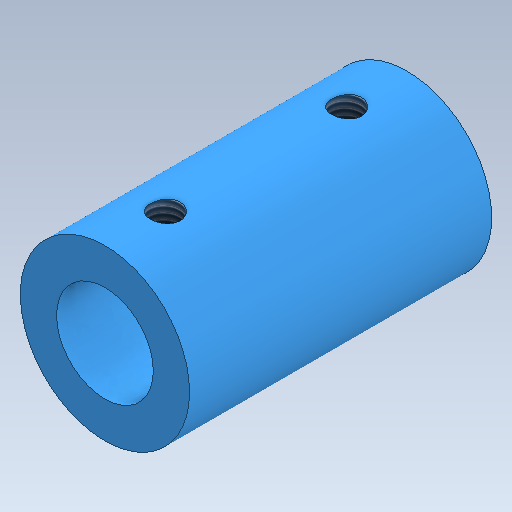
# Autodesk Inventor part: 10-03-05 Hub
Saved by Autodesk Inventor 2020 (Build 240168000, 168)
## iProperties
Created: 2019-10-05
Part Number: 10-03-05 Hub
Material: Generic
Document SubType Name: Modeling
Designer: iuliu
Density: 1 g/cm^3
Appearance: Default(1)
Author: iuliu
Subject: 005
Autodesk Inventor part; units mm, degrees
ref_plane "YZ Plane" through (0, 0, 0) normal (1, 0, 0) x (0, 1, 0)
ref_plane "XZ Plane" through (0, 0, 0) normal (0, 1, 0) x (-1, 0, 0)
ref_plane "XY Plane" through (0, 0, 0) normal (0, 0, 1) x (1, 0, 0)
sketch "Sketch1" plane through (0, 0, 0) normal (0, 0, 1) x (1, 0, 0)
  circle A0 centre (0, 0) radius 7
  dimension "d0" = 14
  constraints: 1 centre point, 1 coincident
  measures "d0" diameter of A0
extrude "Extrusion1" add sketch "Sketch1" along normal blind 25
sketch "Sketch3" plane through (0, 0, 25) normal (0, 0, 1) x (1, 0, 0)
  circle A0 centre (0, 0) radius 7 projected
  constraints: 1 coincident
hole "Hole1" at (0, 0, 25) direction (0, 0, -1) diameter 5 end through all counterbore diameter 8 counterbore depth 12.5
sketch "Sketch4" plane through (0, 0, 0) normal (0, 1, 0) x (-1, 0, 0)
  line L0 (7, 25) -> (-7, 25) projected
  line L1 (7, 0) -> (-7, 0) projected
  point P0 (0, 0)
  point P1 (0, 20)
  point P2 (0, 5)
  dimension "d10" = 5
  dimension "d11" = 5
  constraints: 2 vertical alignment
  measures "d10" distance from line of L0 point (0, 20)
  measures "d11" distance from line of point (0, 5) L1
hole "Hole2" at (0, 0, 20) at (0, 0, 5) direction (0, 1, 0) diameter 2.459 depth 8.8 tip angle 118 thread size "M3x0.5" class "6H" standard "ISO Metric profile"
body "Solid1"
